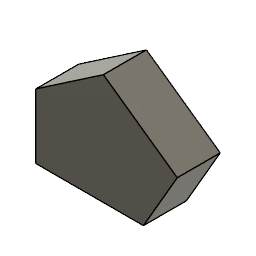
replay (Autodesk Fusion 360 design; units mm, degrees)
Autodesk Fusion 360 part; units mm, degrees
ref_plane "工作平面1" through (0, 0, -9) normal (0, 0, 1) x (1, 0, 0)
sketch "草图1" plane through (0, 0, -9) normal (0, 0, 1) x (1, 0, 0)
  line L0 (15, 10) -> (26, 29)
  line L1 (26, 29) -> (2, 46)
  line L2 (2, 46) -> (-20, 31)
  line L3 (-20, 31) -> (-20, 10)
  line L4 (-20, 10) -> (15, 10)
extrude "拉伸1" add sketch "草图1" along normal blind 14
